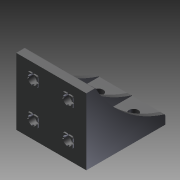
# Autodesk Inventor part: HBLFSDW5h5
Saved by Autodesk Inventor 2011 SP1 (Build 150282100, 282)
## iProperties
Created: 2018-01-07
Part Number: HBLFSDW5h5
Catalog Web Link: www.cadenas.de
Description: HBLFSN5, HBLFSNB5, HBLFSNM5, HBLFSNK5, HBLFSSW5, HBLFSSWB5, HBLFSDW5-Thin Reversal Brackets for Slot Width 6 Frames - For 20, 40mm Sections
Vendor: MISUMI
Document SubType Name: Modeling
Designer: psAdmin
Manufacturer: MISUMI
Mass: 18.5585 g
Surface Area: 106.919 cm^2
Volume: 18.5585 cm^3
Density: 1 g/cm^3
Category: PARTsolutions
Company: MISUMI
Title: HBLFSDW5
Author: Cadenas PARTsolutions
Comments: Thin Reversal Brackets for Slot Width 6 Frames - For 20, 40mm Sections
PSOL_IDENT_0: {$CADENAS_DATA\23d-libs\misumi\metric\38_al_extrusions_blackets\5\hblfsn5.prj},231 {VTYP=3D},{NB=HBL
PSOL_IDENT_1: FSDW5h5},{LINA=HBLFSDW5},{NN=HBLFSN5, HBLFSNB5, HBLFSNM5, HBLFSNK5, HBLFSSW5, HBLFSSWB5, HBLFSDW5},{
PSOL_IDENT_2: DATE=25.12.2017 03:03:09},{GEOMDATE=11.07.2016 08:07:28},{VERSION=},{LINEID=60},{LINESUBID=-1},{WBVA
PSOL_IDENT_3: R=ALT1,ALT2}  {NB=HBLFSDW5h5},{LINA=HBLFSDW5},{KT=3},{PN=HBLFSDW5},{TP=HBLFSDW5},{NOH=2},{NOHV=2},{M
PSOL_IDENT_4: AT=JIS-ADC12},{ST=-},{TYPE=HBLFSDW5},{FEAT=Thin Reversal Bracket},{ALT1=},{ALT2=},{MASS=47},{AB=CBM5
PSOL_IDENT_5: -10},{NOB=8},{AN=HNTT5-5},{NON=8},{AL=2156},{W=40},{H=45},{DP=38},{T=5.0},{HDIS=15},{DPOS=12},{HH1=1
PSOL_IDENT_6: 5},{BOLTX=0.0},{HV1=22},{BOLTY=0.0},{DIA=5.2},{ALT1OPT='','w/o C (Mounting Holes for Cover)','-C','w
PSOL_IDENT_7: ith C (Mounting Holes for Cover)'},{ALT2OPT= '' , 'w/o Set of Applicable Bolt and Nut' , '-SET' , 'w
PSOL_IDENT_8: ith SET (Set of Applicable Bolt and Nut)' , '-SST' , 'with SST (Stainless Steel Set of Applicable Bo
PSOL_IDENT_9: lt and Nut)' , '-SEU' , 'with SEU (Pre-Assembly Fitting Spring Nuts Set of Applicable Bolt and Nut)'
PSOL_IDENT_10: , '-SSU' , 'with SSU (Pre-Assembly Fitting Spring Nuts Stainless Set of Applicable Bolt and Nut)'
PSOL_IDENT_11: , '-SEP' , 'with SEP (Post-Assembly Fitting Spring Nuts Set of Applicable Bolt and Nut)' },{R=1},{R1=
PSOL_IDENT_12: 0.3},{APOSV=0},{VER=1},{PR=3},{TT=0.8},{T1=5}
NN: HBLFSN5, HBLFSNB5, HBLFSNM5, HBLFSNK5, HBLFSSW5, HBLFSSWB5, HBLFSDW5
NT: Thin Reversal Brackets for Slot Width 6 Frames - For 20, 40mm Sections
NB: HBLFSDW5h5
NBSYN: $PN.h5
LINA: HBLFSDW5
PN: HBLFSDW5
TP: HBLFSDW5
MAT: JIS-ADC12
ST: -
FEAT: Thin Reversal Bracket
ALT1: w/o C (Mounting Holes for Cover)
ALT2: w/o Set of Applicable Bolt and Nut
MASS: 47
AB: CBM5-10
NOB: 8
AN: HNTT5-5
NON: 8
AL: 2156
BOLTX: 0.0
BOLTY: 0.0
SUPPLIER: MISUMI
ARTICLENO: HBLFSDW5h5
BOMINFO: HBLFSDW5
CREATOR: CADENAS GmbH
Autodesk Inventor part; units mm, degrees
sketch "Sketch_15" plane through (0, 0, 0) normal (1, 0, 0) x (0, 1, 0)
  line L0 (4.6407, 38) -> (0, 38)
  line L1 (0, 38) -> (0, 0)
  line L2 (0, 0) -> (45, 0)
  line L3 (45, 0) -> (45, 4.5286)
  arc A0 (45, 4.5286) -> (44.6364, 5.3) centre (44, 4.5286) ccw
  line L4 (44.6364, 5.3) -> (5.2771, 37.7714)
  arc A1 (5.2771, 37.7714) -> (4.6407, 38) centre (4.6407, 37) ccw
  constraints: 10 end point, 4 point on circle, 2 centre point
extrude "Extrusion1" add sketch "Sketch_15" along normal mid plane 40
sketch "Sketch_16" plane through (0, 0, 0) normal (1, 0, 0) x (0, 1, 0)
  line L0 (50, 43) -> (5, 43)
  line L1 (5, 43) -> (5, 5)
  line L2 (5, 5) -> (50, 5)
  line L3 (50, 5) -> (50, 43)
  constraints: 8 end point
extrude "Extrusion2" cut sketch "Sketch_16" along normal mid plane 35
sketch "Sketch_21" plane through (0, 0, 0) normal (1, 0, 0) x (0, 1, 0)
  line L0 (4.6407, 38) -> (0, 38)
  line L1 (0, 38) -> (0, 0)
  line L2 (0, 0) -> (45, 0)
  line L3 (45, 0) -> (45, 4.5286)
  arc A0 (45, 4.5286) -> (44.6364, 5.3) centre (44, 4.5286) ccw
  line L4 (44.6364, 5.3) -> (5.2771, 37.7714)
  arc A1 (5.2771, 37.7714) -> (4.6407, 38) centre (4.6407, 37) ccw
  constraints: 10 end point, 4 point on circle, 2 centre point
extrude "Extrusion3" add sketch "Sketch_21" along normal mid plane 2.5
sketch "Sketch_28" plane through (0, 0, 0) normal (1, 0, 0) x (0, 1, 0)
  arc A0 (5.2771, 37.7714) -> (44.6364, 5.3) centre (64.787, 69.8148) ccw
  line L0 (44.6364, 5.3) -> (5.2771, 37.7714)
  constraints: 2 end point, 2 point on circle, 1 centre point
extrude "Extrusion4" cut sketch "Sketch_28" along normal mid plane 40
sketch "Sketch_22_ALT_Drilling_1" plane through (0, 0, 0) normal (0, 1, 0) x (-1, 0, 0)
  circle A0 centre (10, 10) radius 2.6
  constraints: 1 centre point
extrude "Extrusion5" cut sketch "Sketch_22_ALT_Drilling_1" along normal blind 5
sketch "Pattern_3_SKETCH_1" plane through (20, 0, 0) normal (0, 1, 0) x (1, 0, 0)
  circle A0 centre (-10, -10) radius 2.6
  constraints: 1 centre point
sketch "Pattern_3_SKETCH_2" plane through (0, 0, 20) normal (0, 1, 0) x (1, 0, 0)
  circle A0 centre (-10, -10) radius 2.6
  constraints: 1 centre point
sketch "Pattern_3_SKETCH_3" plane through (20, 0, 20) normal (0, 1, 0) x (1, 0, 0)
  circle A0 centre (-10, -10) radius 2.6
  constraints: 1 centre point
extrude "Extrusion6" cut sketch "Pattern_3_SKETCH_1" along normal blind 5
extrude "Extrusion7" cut sketch "Pattern_3_SKETCH_2" along normal blind 5
extrude "Extrusion8" cut sketch "Pattern_3_SKETCH_3" along normal blind 5
sketch "Sketch_24_ALT_Drilling_2" plane through (0, 0, 0) normal (0, 0, 1) x (1, 0, 0)
  circle A0 centre (-10, 22) radius 2.6
  constraints: 1 centre point
extrude "Extrusion9" cut sketch "Sketch_24_ALT_Drilling_2" along normal blind 5
sketch "Pattern_4_SKETCH_1" plane through (20, 0, 0) normal (0, 0, 1) x (1, 0, 0)
  circle A0 centre (-10, 22) radius 2.6
  constraints: 1 centre point
sketch "Pattern_4_SKETCH_2" plane through (0, 15, 0) normal (0, 0, 1) x (1, 0, 0)
  circle A0 centre (-10, 22) radius 2.6
  constraints: 1 centre point
sketch "Pattern_4_SKETCH_3" plane through (20, 15, 0) normal (0, 0, 1) x (1, 0, 0)
  circle A0 centre (-10, 22) radius 2.6
  constraints: 1 centre point
extrude "Extrusion10" cut sketch "Pattern_4_SKETCH_1" along normal blind 5
extrude "Extrusion11" cut sketch "Pattern_4_SKETCH_2" along normal blind 5
extrude "Extrusion12" cut sketch "Pattern_4_SKETCH_3" along normal blind 5
sketch "Sketch_1" plane through (0, 0, 0) normal (0, 1, 0) x (-1, 0, 0)
  line L0 (20, 38) -> (-20, 38)
  line L1 (-20, 38) -> (-20, 0)
  line L2 (-20, 0) -> (20, 0)
  line L3 (20, 0) -> (20, 38)
  constraints: 8 end point
extrude "Extrusion13" add sketch "Sketch_1" against normal blind 0.8
sketch "Sketch_10" plane through (0, 0, 0) normal (0, 0, 1) x (1, 0, 0)
  line L0 (-20, 45) -> (-20, 0)
  line L1 (-20, 0) -> (20, 0)
  line L2 (20, 0) -> (20, 45)
  line L3 (20, 45) -> (-20, 45)
  constraints: 8 end point
extrude "Extrusion14" add sketch "Sketch_10" against normal blind 0.8
sketch "Sketch_14" plane through (0, 0, 0) normal (0, 1, 0) x (-1, 0, 0)
  line L0 (20, 38) -> (-20, 38)
  line L1 (-20, 38) -> (-20, 0)
  line L2 (-20, 0) -> (20, 0)
  line L3 (20, 0) -> (20, 38)
  arc A0 (-12.5515, 9.5) -> (-10.5, 7.4485) centre (-10, 10) ccw
  line L4 (-12.5515, 9.5) -> (-13, 9.5)
  line L5 (-13, 9.5) -> (-13, 8)
  arc A1 (-13, 8) -> (-12, 7) centre (-12, 8) ccw
  line L6 (-12, 7) -> (-10.5, 7)
  line L7 (-10.5, 7) -> (-10.5, 7.4485)
  line L8 (-10.5, 12.5515) -> (-10.5, 13)
  line L9 (-10.5, 13) -> (-12, 13)
  arc A2 (-12, 13) -> (-13, 12) centre (-12, 12) ccw
  line L10 (-13, 12) -> (-13, 10.5)
  line L11 (-13, 10.5) -> (-12.5515, 10.5)
  arc A3 (-10.5, 12.5515) -> (-12.5515, 10.5) centre (-10, 10) ccw
  arc A4 (-12.5515, 29.5) -> (-10.5, 27.4485) centre (-10, 30) ccw
  line L12 (-12.5515, 29.5) -> (-13, 29.5)
  line L13 (-13, 29.5) -> (-13, 28)
  arc A5 (-13, 28) -> (-12, 27) centre (-12, 28) ccw
  line L14 (-12, 27) -> (-10.5, 27)
  line L15 (-10.5, 27) -> (-10.5, 27.4485)
  line L16 (-10.5, 32.5515) -> (-10.5, 33)
  line L17 (-10.5, 33) -> (-12, 33)
  arc A6 (-12, 33) -> (-13, 32) centre (-12, 32) ccw
  line L18 (-13, 32) -> (-13, 30.5)
  line L19 (-13, 30.5) -> (-12.5515, 30.5)
  arc A7 (-10.5, 32.5515) -> (-12.5515, 30.5) centre (-10, 30) ccw
  line L20 (-7, 8) -> (-7, 9.5)
  line L21 (-7, 9.5) -> (-7.4485, 9.5)
  arc A8 (-9.5, 7.4485) -> (-7.4485, 9.5) centre (-10, 10) ccw
  line L22 (-9.5, 7.4485) -> (-9.5, 7)
  line L23 (-9.5, 7) -> (-8, 7)
  arc A9 (-8, 7) -> (-7, 8) centre (-8, 8) ccw
  line L24 (-7, 10.5) -> (-7, 12)
  arc A10 (-7, 12) -> (-8, 13) centre (-8, 12) ccw
  line L25 (-8, 13) -> (-9.5, 13)
  line L26 (-9.5, 13) -> (-9.5, 12.5515)
  arc A11 (-7.4485, 10.5) -> (-9.5, 12.5515) centre (-10, 10) ccw
  line L27 (-7.4485, 10.5) -> (-7, 10.5)
  line L28 (-7, 28) -> (-7, 29.5)
  line L29 (-7, 29.5) -> (-7.4485, 29.5)
  arc A12 (-9.5, 27.4485) -> (-7.4485, 29.5) centre (-10, 30) ccw
  line L30 (-9.5, 27.4485) -> (-9.5, 27)
  line L31 (-9.5, 27) -> (-8, 27)
  arc A13 (-8, 27) -> (-7, 28) centre (-8, 28) ccw
  line L32 (-7, 30.5) -> (-7, 32)
  arc A14 (-7, 32) -> (-8, 33) centre (-8, 32) ccw
  line L33 (-8, 33) -> (-9.5, 33)
  line L34 (-9.5, 33) -> (-9.5, 32.5515)
  arc A15 (-7.4485, 30.5) -> (-9.5, 32.5515) centre (-10, 30) ccw
  line L35 (-7.4485, 30.5) -> (-7, 30.5)
  arc A16 (7.4485, 9.5) -> (9.5, 7.4485) centre (10, 10) ccw
  line L36 (7.4485, 9.5) -> (7, 9.5)
  line L37 (7, 9.5) -> (7, 8)
  arc A17 (7, 8) -> (8, 7) centre (8, 8) ccw
  line L38 (8, 7) -> (9.5, 7)
  line L39 (9.5, 7) -> (9.5, 7.4485)
  line L40 (9.5, 12.5515) -> (9.5, 13)
  line L41 (9.5, 13) -> (8, 13)
  arc A18 (8, 13) -> (7, 12) centre (8, 12) ccw
  line L42 (7, 12) -> (7, 10.5)
  line L43 (7, 10.5) -> (7.4485, 10.5)
  arc A19 (9.5, 12.5515) -> (7.4485, 10.5) centre (10, 10) ccw
  arc A20 (7.4485, 29.5) -> (9.5, 27.4485) centre (10, 30) ccw
  line L44 (7.4485, 29.5) -> (7, 29.5)
  line L45 (7, 29.5) -> (7, 28)
  arc A21 (7, 28) -> (8, 27) centre (8, 28) ccw
  line L46 (8, 27) -> (9.5, 27)
  line L47 (9.5, 27) -> (9.5, 27.4485)
  line L48 (9.5, 32.5515) -> (9.5, 33)
  line L49 (9.5, 33) -> (8, 33)
  arc A22 (8, 33) -> (7, 32) centre (8, 32) ccw
  line L50 (7, 32) -> (7, 30.5)
  line L51 (7, 30.5) -> (7.4485, 30.5)
  arc A23 (9.5, 32.5515) -> (7.4485, 30.5) centre (10, 30) ccw
  line L52 (13, 8) -> (13, 9.5)
  line L53 (13, 9.5) -> (12.5515, 9.5)
  arc A24 (10.5, 7.4485) -> (12.5515, 9.5) centre (10, 10) ccw
  line L54 (10.5, 7.4485) -> (10.5, 7)
  line L55 (10.5, 7) -> (12, 7)
  arc A25 (12, 7) -> (13, 8) centre (12, 8) ccw
  line L56 (13, 10.5) -> (13, 12)
  arc A26 (13, 12) -> (12, 13) centre (12, 12) ccw
  line L57 (12, 13) -> (10.5, 13)
  line L58 (10.5, 13) -> (10.5, 12.5515)
  arc A27 (12.5515, 10.5) -> (10.5, 12.5515) centre (10, 10) ccw
  line L59 (12.5515, 10.5) -> (13, 10.5)
  line L60 (13, 28) -> (13, 29.5)
  line L61 (13, 29.5) -> (12.5515, 29.5)
  arc A28 (10.5, 27.4485) -> (12.5515, 29.5) centre (10, 30) ccw
  line L62 (10.5, 27.4485) -> (10.5, 27)
  line L63 (10.5, 27) -> (12, 27)
  arc A29 (12, 27) -> (13, 28) centre (12, 28) ccw
  line L64 (13, 30.5) -> (13, 32)
  arc A30 (13, 32) -> (12, 33) centre (12, 32) ccw
  line L65 (12, 33) -> (10.5, 33)
  line L66 (10.5, 33) -> (10.5, 32.5515)
  arc A31 (12.5515, 30.5) -> (10.5, 32.5515) centre (10, 30) ccw
  line L67 (12.5515, 30.5) -> (13, 30.5)
  constraints: 136 end point, 64 point on circle, 32 centre point
extrude "Extrusion15" cut sketch "Sketch_14" against normal blind 0.8
sketch "Sketch_27" plane through (0, 0, 0) normal (0, 0, 1) x (1, 0, 0)
  line L0 (-20, 0) -> (20, 0)
  line L1 (20, 0) -> (20, 45)
  line L2 (20, 45) -> (-20, 45)
  line L3 (-20, 45) -> (-20, 0)
  line L4 (7, 7.7) -> (7, 3.3)
  arc A0 (7, 3.3) -> (7.3, 3) centre (7.3, 3.3) ccw
  line L5 (7.3, 3) -> (12.7, 3)
  arc A1 (12.7, 3) -> (13, 3.3) centre (12.7, 3.3) ccw
  line L6 (13, 3.3) -> (13, 7.7)
  arc A2 (13, 7.7) -> (12.7, 8) centre (12.7, 7.7) ccw
  line L7 (12.7, 8) -> (7.3, 8)
  arc A3 (7.3, 8) -> (7, 7.7) centre (7.3, 7.7) ccw
  line L8 (7, 32.7) -> (7, 27.3)
  arc A4 (7, 27.3) -> (7.3, 27) centre (7.3, 27.3) ccw
  line L9 (7.3, 27) -> (12.7, 27)
  arc A5 (12.7, 27) -> (13, 27.3) centre (12.7, 27.3) ccw
  line L10 (13, 27.3) -> (13, 32.7)
  arc A6 (13, 32.7) -> (12.7, 33) centre (12.7, 32.7) ccw
  line L11 (12.7, 33) -> (7.3, 33)
  arc A7 (7.3, 33) -> (7, 32.7) centre (7.3, 32.7) ccw
  line L12 (-13, 7.7) -> (-13, 3.3)
  arc A8 (-13, 3.3) -> (-12.7, 3) centre (-12.7, 3.3) ccw
  line L13 (-12.7, 3) -> (-7.3, 3)
  arc A9 (-7.3, 3) -> (-7, 3.3) centre (-7.3, 3.3) ccw
  line L14 (-7, 3.3) -> (-7, 7.7)
  arc A10 (-7, 7.7) -> (-7.3, 8) centre (-7.3, 7.7) ccw
  line L15 (-7.3, 8) -> (-12.7, 8)
  arc A11 (-12.7, 8) -> (-13, 7.7) centre (-12.7, 7.7) ccw
  line L16 (-13, 32.7) -> (-13, 27.3)
  arc A12 (-13, 27.3) -> (-12.7, 27) centre (-12.7, 27.3) ccw
  line L17 (-12.7, 27) -> (-7.3, 27)
  arc A13 (-7.3, 27) -> (-7, 27.3) centre (-7.3, 27.3) ccw
  line L18 (-7, 27.3) -> (-7, 32.7)
  arc A14 (-7, 32.7) -> (-7.3, 33) centre (-7.3, 32.7) ccw
  line L19 (-7.3, 33) -> (-12.7, 33)
  arc A15 (-12.7, 33) -> (-13, 32.7) centre (-12.7, 32.7) ccw
  constraints: 40 end point, 32 point on circle, 16 centre point
extrude "Extrusion16" cut sketch "Sketch_27" against normal blind 1.25
ref_plane "4_bolt_row_12_1_XY" through (-10, 22, 5) normal (0, 0, 1) x (1, 0, 0)
ref_plane "4_bolt_row_12_1_YZ" through (-10, 22, 5) normal (1, 0, 0) x (0, 1, 0)
ref_plane "4_bolt_row_12_1_ZX" through (-10, 22, 5) normal (0, 1, 0) x (0, 0, 1)
ref_plane "4_bolt_row_12_2_XY" through (10, 22, 5) normal (0, 0, 1) x (1, 0, 0)
ref_plane "4_bolt_row_12_2_YZ" through (10, 22, 5) normal (1, 0, 0) x (0, 1, 0)
ref_plane "4_bolt_row_12_2_ZX" through (10, 22, 5) normal (0, 1, 0) x (0, 0, 1)
ref_plane "4_bolt_row_12_3_XY" through (-10, 37, 5) normal (0, 0, 1) x (1, 0, 0)
ref_plane "4_bolt_row_12_3_YZ" through (-10, 37, 5) normal (1, 0, 0) x (0, 1, 0)
ref_plane "4_bolt_row_12_3_ZX" through (-10, 37, 5) normal (0, 1, 0) x (0, 0, 1)
ref_plane "4_bolt_row_12_4_XY" through (10, 37, 5) normal (0, 0, 1) x (1, 0, 0)
ref_plane "4_bolt_row_12_4_YZ" through (10, 37, 5) normal (1, 0, 0) x (0, 1, 0)
ref_plane "4_bolt_row_12_4_ZX" through (10, 37, 5) normal (0, 1, 0) x (0, 0, 1)
ref_plane "4_hole_row_12_base_1_XY" through (-10, 5, 10) normal (0, 1, 0) x (1, 0, 0)
ref_plane "4_hole_row_12_base_1_YZ" through (-10, 5, 10) normal (1, 0, 0) x (0, 0, -1)
ref_plane "4_hole_row_12_base_1_ZX" through (-10, 5, 10) normal (0, 0, -1) x (0, 1, 0)
ref_plane "4_hole_row_12_base_2_XY" through (10, 5, 10) normal (0, 1, 0) x (1, 0, 0)
ref_plane "4_hole_row_12_base_2_YZ" through (10, 5, 10) normal (1, 0, 0) x (0, 0, -1)
ref_plane "4_hole_row_12_base_2_ZX" through (10, 5, 10) normal (0, 0, -1) x (0, 1, 0)
ref_plane "4_hole_row_12_base_3_XY" through (-10, 5, 30) normal (0, 1, 0) x (1, 0, 0)
ref_plane "4_hole_row_12_base_3_YZ" through (-10, 5, 30) normal (1, 0, 0) x (0, 0, -1)
ref_plane "4_hole_row_12_base_3_ZX" through (-10, 5, 30) normal (0, 0, -1) x (0, 1, 0)
ref_plane "4_hole_row_12_base_4_XY" through (10, 5, 30) normal (0, 1, 0) x (1, 0, 0)
ref_plane "4_hole_row_12_base_4_YZ" through (10, 5, 30) normal (1, 0, 0) x (0, 0, -1)
ref_plane "4_hole_row_12_base_4_ZX" through (10, 5, 30) normal (0, 0, -1) x (0, 1, 0)
ref_plane "4_nut_row_12_1_XY" through (-10, 22, -2) normal (0, 0, 1) x (1, 0, 0)
ref_plane "4_nut_row_12_1_YZ" through (-10, 22, -2) normal (1, 0, 0) x (0, 1, 0)
ref_plane "4_nut_row_12_1_ZX" through (-10, 22, -2) normal (0, 1, 0) x (0, 0, 1)
ref_plane "4_nut_row_12_2_XY" through (10, 22, -2) normal (0, 0, 1) x (1, 0, 0)
ref_plane "4_nut_row_12_2_YZ" through (10, 22, -2) normal (1, 0, 0) x (0, 1, 0)
ref_plane "4_nut_row_12_2_ZX" through (10, 22, -2) normal (0, 1, 0) x (0, 0, 1)
ref_plane "4_nut_row_12_3_XY" through (-10, 37, -2) normal (0, 0, 1) x (1, 0, 0)
ref_plane "4_nut_row_12_3_YZ" through (-10, 37, -2) normal (1, 0, 0) x (0, 1, 0)
ref_plane "4_nut_row_12_3_ZX" through (-10, 37, -2) normal (0, 1, 0) x (0, 0, 1)
ref_plane "4_nut_row_12_4_XY" through (10, 37, -2) normal (0, 0, 1) x (1, 0, 0)
ref_plane "4_nut_row_12_4_YZ" through (10, 37, -2) normal (1, 0, 0) x (0, 1, 0)
ref_plane "4_nut_row_12_4_ZX" through (10, 37, -2) normal (0, 1, 0) x (0, 0, 1)
ref_plane "4_nut_row_12_base_1_XY" through (-10, -2, 10) normal (0, 1, 0) x (1, 0, 0)
ref_plane "4_nut_row_12_base_1_YZ" through (-10, -2, 10) normal (1, 0, 0) x (0, 0, -1)
ref_plane "4_nut_row_12_base_1_ZX" through (-10, -2, 10) normal (0, 0, -1) x (0, 1, 0)
ref_plane "4_nut_row_12_base_2_XY" through (10, -2, 10) normal (0, 1, 0) x (1, 0, 0)
ref_plane "4_nut_row_12_base_2_YZ" through (10, -2, 10) normal (1, 0, 0) x (0, 0, -1)
ref_plane "4_nut_row_12_base_2_ZX" through (10, -2, 10) normal (0, 0, -1) x (0, 1, 0)
ref_plane "4_nut_row_12_base_3_XY" through (-10, -2, 30) normal (0, 1, 0) x (1, 0, 0)
ref_plane "4_nut_row_12_base_3_YZ" through (-10, -2, 30) normal (1, 0, 0) x (0, 0, -1)
ref_plane "4_nut_row_12_base_3_ZX" through (-10, -2, 30) normal (0, 0, -1) x (0, 1, 0)
ref_plane "4_nut_row_12_base_4_XY" through (10, -2, 30) normal (0, 1, 0) x (1, 0, 0)
ref_plane "4_nut_row_12_base_4_YZ" through (10, -2, 30) normal (1, 0, 0) x (0, 0, -1)
ref_plane "4_nut_row_12_base_4_ZX" through (10, -2, 30) normal (0, 0, -1) x (0, 1, 0)
ref_plane "bracket_to_bolt_XY" through (1, 22, 0) normal (0, 0, 1) x (1, 0, 0)
ref_plane "bracket_to_bolt_YZ" through (1, 22, 0) normal (1, 0, 0) x (0, 1, 0)
ref_plane "bracket_to_bolt_ZX" through (1, 22, 0) normal (0, 1, 0) x (0, 0, 1)
ref_plane "bracket_to_dummy_XY" through (0, 0, 0) normal (0, 1, 0) x (1, 0, 0)
ref_plane "bracket_to_dummy_YZ" through (0, 0, 0) normal (1, 0, 0) x (0, 0, -1)
ref_plane "bracket_to_dummy_ZX" through (0, 0, 0) normal (0, 0, -1) x (0, 1, 0)
body "Solid1"
